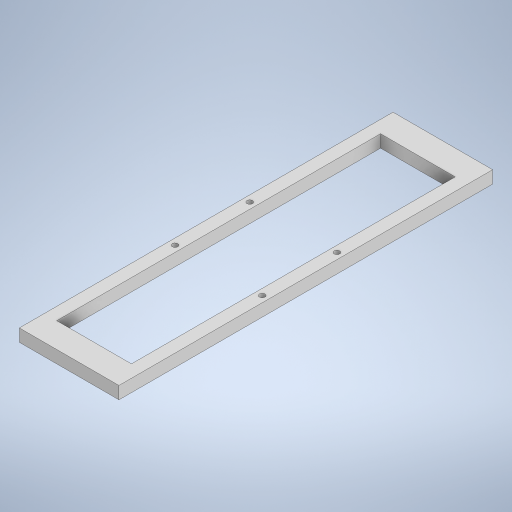
# Autodesk Inventor part: 발판보강지지대2
Saved by Autodesk Inventor 2024 (Build 280153000, 153)
## iProperties
Created: 2024-06-07
Part Number: 발판보강지지대2
Material: 일반
Document SubType Name: Modeling
Designer: kkamin5
Density: 1 g/cm^3
Appearance: 기본값
Author: kkamin5
Autodesk Inventor part; units mm, degrees
ref_plane "YZ Plane" through (0, 0, 0) normal (1, 0, 0) x (0, 1, 0)
ref_plane "XZ Plane" through (0, 0, 0) normal (0, 1, 0) x (-1, 0, 0)
ref_plane "XY Plane" through (0, 0, 0) normal (0, 0, 1) x (1, 0, 0)
sketch "스케치1" plane through (0, 0, 0) normal (0, 1, 0) x (-1, 0, 0)
  line L0 (-40, 150) -> (40, 150)
  line L1 (40, 150) -> (40, -150)
  line L2 (40, -150) -> (-40, -150)
  line L3 (-40, -150) -> (-40, 150)
  line L4 (-40, 150) -> (40, -150) construction
  line L5 (40, 150) -> (-40, -150) construction
  line L6 (-30, 130) -> (30, 130)
  line L7 (30, 130) -> (30, -130)
  line L8 (30, -130) -> (-30, -130)
  line L9 (-30, -130) -> (-30, 130)
  line L10 (-30, 130) -> (30, -130) construction
  line L11 (30, 130) -> (-30, -130) construction
  circle A0 centre (35, 30) radius 2.25
  circle A1 centre (35, -30) radius 2.25
  circle A2 centre (-35, -30) radius 2.25
  circle A3 centre (-35, 30) radius 2.25
  point P0 (0, 0)
  dimension "d0" = 80
  dimension "d1" = 300
  dimension "d2" = 60
  dimension "d3" = 260
  dimension "d4" = 0
  dimension "d5" = 0
  dimension "d6" = 0
  dimension "d7" = 0
  dimension "d8" = 70
  dimension "d9" = 35
  dimension "d10" = 60
  dimension "d11" = 30
  dimension "d12" = 4.5
  dimension "d13" = 4.5
  dimension "d14" = 4.5
  dimension "d15" = 4.5
  constraints: 24 end point, 4 centre point, 4 coincident, 4 midpoint, 4 parallel, 2 horizontal, 2 perpendicular
  measures "d0" distance of L1.end L2.end
  measures "d1" distance of L0.end L1.end
  measures "d2" distance of L7.end L8.end
  measures "d3" distance of L6.end L7.end
  measures "d4" horizontal distance of point (-35, -30) point (-35, 30)
  measures "d5" vertical distance of point (35, 30) point (-35, 30)
  measures "d6" vertical distance of point (35, -30) point (-35, -30)
  measures "d7" horizontal distance of point (35, 30) point (35, -30)
  measures "d8" distance of point (35, 30) point (-35, 30)
  measures "d9" horizontal distance of point (0, 0) point (35, 30)
  measures "d10" distance of point (-35, 30) point (-35, -30)
  measures "d11" vertical distance of point (0, 0) point (-35, 30)
  measures "d12" diameter of A0
  measures "d13" diameter of A1
  measures "d14" diameter of A2
  measures "d15" diameter of A3
extrude "돌출1" add sketch "스케치1" along normal blind 10
equation "\"d9\" = 0.5 * d8"
equation "\"d11\" = 0.5 * d10"
